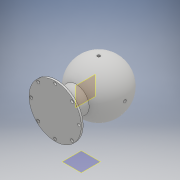
# Autodesk Inventor part: Rotula_dron_p1
Saved by Autodesk Inventor 2017 (Build 210142000, 142)
## iProperties
Created: 2017-09-09
Part Number: Rotula_dron_p1
Material: Generic
Document SubType Name: Modeling
Designer: penacionación
Density: 1 g/cm^3
Appearance: Default
Author: penacionación
Autodesk Inventor part; units mm, degrees
ref_plane "YZ Plane" through (0, 0, 0) normal (1, 0, 0) x (0, 1, 0)
ref_plane "XZ Plane" through (0, 0, 0) normal (0, 1, 0) x (-1, 0, 0)
ref_plane "XY Plane" through (0, 0, 0) normal (0, 0, 1) x (1, 0, 0)
sketch "Sketch1" plane through (0, 0, 0) normal (0, 0, 1) x (1, 0, 0)
  arc A0 (15, -25.9808) -> (0, 30) centre (0, 0) ccw
  line L0 (0, 0) -> (0, -30)
  line L1 (0, 0) -> (0, 30)
  line L2 (0, -30) -> (0, -50)
  line L3 (0, -50) -> (30, -50)
  arc A1 (15, -25.9808) -> (24.3562, -47.7564) centre (34.4808, -30.5084) ccw
  line L4 (24.8625, -47.894) -> (30, -47.894)
  line L5 (30, -47.894) -> (30, -50)
  arc A2 (24.3562, -47.7564) -> (24.8625, -47.894) centre (24.8625, -46.894) ccw
  point P0 (24.5944, -47.894)
  dimension "d0" = 60
  dimension "d3" = 20
  dimension "d4" = 30
  dimension "d5" = 20
  dimension "d6" = 1
  constraints: 12 end point, 7 point on circle, 3 centre point, 2 perpendicular, 2 point on line, 2 tangent, 2 vertical, 1 coincident, 1 horizontal
  measures "d0" diameter of A0
  measures "d3" distance of L0.end L2.end
  measures "d4" distance of L2.end L3.end
  measures "d5" radius of A1
  measures "d6" radius of A2
revolve "Revolution1" add sketch "Sketch1" angle 360 about axis through (0, 0, 0) along (0, -1, 0)
sketch "Sketch2" plane through (0, -50, 0) normal (0, -1, 0) x (1, 0, 0)
  circle A0 centre (0, 0) radius 24.8625
  circle A1 centre (0, 0) radius 30 projected
  line L0 (0, 30) -> (0, 24.8625)
  circle A2 centre (0, 27.4312) radius 1.6
  line L1 (17.5804, 17.5804) -> (21.2132, 21.2132)
  line L2 (0, 0) -> (0, 24.8625)
  circle A3 centre (19.3968, 19.3968) radius 1.76
  line L3 (24.8625, 0) -> (30, 0)
  circle A4 centre (27.4312, 0) radius 1.6
  circle A5 centre (0, 27.4312) radius 1.6
  circle A6 centre (0, 27.4312) radius 1.6
  circle A7 centre (-19.3968, 19.3968) radius 1.76
  circle A8 centre (-27.4312, 0) radius 1.6
  line L4 (0, 0) -> (24.8625, 0)
  circle A9 centre (0, -27.4312) radius 1.6
  circle A10 centre (19.3968, -19.3968) radius 1.76
  circle A11 centre (27.4312, 0) radius 1.6
  circle A12 centre (-19.3968, -19.3968) radius 1.76
  circle A13 centre (-27.4312, 0) radius 1.6
  dimension "d8" = 3.2
  dimension "d9" = 45
  dimension "d10" = 3.52
  dimension "d11" = 3.2
  constraints: 13 centre point, 10 end point, 6 point on circle, 5 symmetric about line, 3 midpoint, 2 horizontal, 2 vertical, 1 coincident, 9 other
  measures "d8" diameter of A2
  measures "d9" angle of L2 L1
  measures "d10" diameter of A3
  measures "d11" diameter of A4
extrude "Extrusion1" cut sketch "Sketch2" against normal blind 10 contours A4 L3 | L3 A4 | A3 L1 | L1 A3 | A2 L0 | L0 A2 | A7 | A8 | A9 | A10 | A12
ref_plane "Work Plane1" through (30, -50, -35.2597) normal (0, 0, -1) x (-1, 0, 0)
sketch "Sketch4" plane through (30, -50, -35.2597) normal (0, 0, -1) x (-1, 0, 0)
  circle A0 centre (30, 50) radius 30
  circle A1 centre (30, 50) radius 1.6
  dimension "d16" = 60
  dimension "d17" = 3.2
  constraints: 2 centre point, 2 coincident
  measures "d16" diameter of A0
  measures "d17" diameter of A1
extrude "Extrusion3" cut sketch "Sketch4" against normal blind 73.75 contours A1
ref_plane "Work Plane2" through (34.8176, -50, 37.4918) normal (1, 0, 0) x (0, 0, -1)
sketch "Sketch6" plane through (34.8176, -50, 37.4918) normal (1, 0, 0) x (0, 0, -1)
  circle A0 centre (37.4918, 50) radius 30
  circle A1 centre (37.4918, 50) radius 1.6
  dimension "d22" = 60
  dimension "d23" = 3.2
  constraints: 2 centre point, 2 coincident
  measures "d22" diameter of A0
  measures "d23" diameter of A1
extrude "Extrusion5" cut sketch "Sketch6" against normal blind 74.75 contours A1
body "Solid1"
